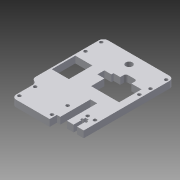
# Autodesk Inventor part: yCarTop
Saved by Autodesk Inventor 2013 (Build 170138000, 138)
## iProperties
Created: 2015-01-14
Part Number: yCarTop
Material: Generic
Document SubType Name: Modeling
Designer: dzban
Density: 1 g/cm^3
Author: dzban
Autodesk Inventor part; units mm, degrees
ref_plane "YZ Plane" through (0, 0, 0) normal (1, 0, 0) x (0, 1, 0)
ref_plane "XZ Plane" through (0, 0, 0) normal (0, 1, 0) x (-1, 0, 0)
ref_plane "XY Plane" through (0, 0, 0) normal (0, 0, 1) x (1, 0, 0)
sketch "Sketch1" plane through (0, 0, 0) normal (0, 0, 1) x (1, 0, 0)
  line L0 (-31, 44) -> (-31, 55.9)
  line L1 (-31, 55.9) -> (-37.25, 55.9)
  line L2 (-37.25, 55.9) -> (-37.25, 62.1)
  line L3 (-37.25, 62.1) -> (-31, 62.1)
  line L4 (-31, 62.1) -> (-31, 64)
  line L5 (-31, 64) -> (-25, 64)
  line L6 (-25, 64) -> (-25, 67)
  arc A0 (-23, 69) -> (-25, 67) centre (-23, 67) ccw
  line L7 (-23, 69) -> (-17, 69)
  arc A1 (-15, 67) -> (-17, 69) centre (-17, 67) ccw
  line L8 (-15, 67) -> (-15, 64)
  line L9 (-15, 64) -> (-6, 64)
  line L10 (-6, 64) -> (-6, 44)
  line L11 (-6, 44) -> (-31, 44)
  line L12 (-61.6, 39.5) -> (-61.6, 60.5)
  line L13 (-61.6, 60.5) -> (-46.4, 60.5)
  line L14 (-46.4, 60.5) -> (-46.4, 39.5)
  line L15 (-46.4, 39.5) -> (-61.6, 39.5)
  circle A2 centre (-30.9, 77.8) radius 3
  circle A3 centre (-3, 59) radius 1.5
  circle A4 centre (-26.5, 18.5) radius 1.5
  circle A5 centre (-26.5, 4.5) radius 1.5
  circle A6 centre (-55.5, 4.5) radius 1.5
  circle A7 centre (-55.5, 18.5) radius 1.5
  circle A8 centre (-3, 19.5) radius 1.5
  circle A9 centre (-9.5, 19.5) radius 1.5
  circle A10 centre (-60.5, 68.5) radius 1.5
  circle A11 centre (-60.5, 82.5) radius 1.5
  circle A12 centre (-2.5, 82.5) radius 1.5
  circle A13 centre (-2.5, 68.5) radius 1.5
  arc A14 (0, 83) -> (-4, 87) centre (-4, 83) ccw
  line L16 (-4, 87) -> (-59, 87)
  arc A15 (-59, 87) -> (-63, 83) centre (-59, 83) ccw
  line L17 (-63, 83) -> (-63, 26.3448)
  arc A16 (-63, 26.3448) -> (-60.5004, 22.6368) centre (-59, 26.3448) ccw
  arc A17 (-58.0008, 18.9289) -> (-60.5004, 22.6368) centre (-62.0008, 18.9289) ccw
  line L18 (-58.0008, 18.9289) -> (-58.0008, 4)
  arc A18 (-58.0008, 4) -> (-54.0008, 0) centre (-54.0008, 4) ccw
  line L19 (-54.0008, 0) -> (-24, 0)
  line L20 (-24, 0) -> (-24, 6.4)
  line L21 (-24, 6.4) -> (-21, 6.4)
  line L22 (-21, 6.4) -> (-21, 33.4)
  line L23 (-21, 33.4) -> (-15, 33.4)
  line L24 (-15, 33.4) -> (-15, 6.4)
  line L25 (-15, 6.4) -> (-9, 6.4)
  line L26 (-9, 6.4) -> (-9, 13.4)
  line L27 (-9, 13.4) -> (-10.25, 13.4)
  line L28 (-10.25, 13.4) -> (-10.25, 15.2)
  line L29 (-10.25, 15.2) -> (-9, 15.2)
  line L30 (-9, 15.2) -> (-9, 17)
  line L31 (-9, 17) -> (-6, 17)
  line L32 (-6, 17) -> (-6, 15.2)
  line L33 (-6, 15.2) -> (-4.75, 15.2)
  line L34 (-4.75, 15.2) -> (-4.75, 13.4)
  line L35 (-4.75, 13.4) -> (-6, 13.4)
  line L36 (-6, 13.4) -> (-6, 6.4)
  line L37 (-6, 6.4) -> (0, 6.4)
  line L38 (0, 6.4) -> (0, 83)
  point P0 (0, 0)
  point P1 (0, 0)
  constraints: 78 end point, 19 centre point, 14 point on circle
extrude "Extrusion1" add sketch "Sketch1" along normal blind 6
body "Solid1"
